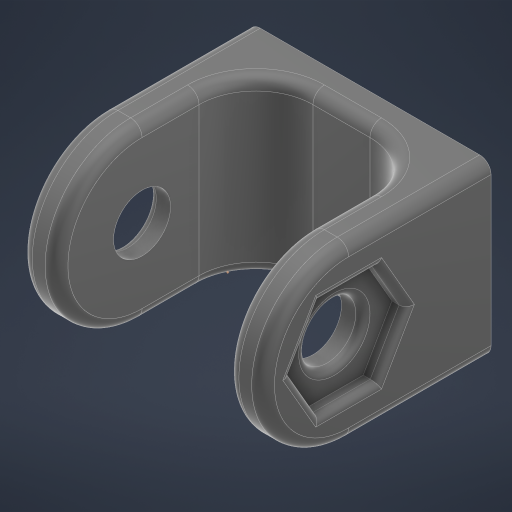
# Autodesk Inventor part: board_box_holder
Saved by Autodesk Inventor 2023 (Build 270158030, 158C)
## iProperties
Created: 2022-07-16
Part Number: board_box_holder
Material: Thermoplastic Resin
Document SubType Name: Modeling
Designer: Norbert Ligas
Density: 1.28 g/cm^3
Appearance: Smooth - Black
bar_holder_bar_diameter: 8,000 mm
bar_holder_wall_thickness: 2,000 mm
bar_holder_holder_depth: 20,000 mm
bar_holder_holder_length: 22,000 mm
bar_holder_screw_diameter: 4,000 mm
bar_holder_screw_to_bar_distance: 0,500 mm
nut_width: 7,000 mm
screw_head_diameter: 7,000 mm
bar_connector_width: 2,500 mm
bar_connector_screw_depth: 1,000 mm
bar_connector_bar_holder_width: 12,000 mm
bar_connector_length_from_screw_center_to_edge: 6,000 mm
bar_connector_min_length_from_screw_center_to_box: 6,000 mm
bar_connector_min_length_from_screw_center_to_box_margin: 2,000 mm
bar_connector_length_from_screw_center_to_box: 8,000 mm
d32: 12,000 mm
d33: 2,500 mm
d35: 6,000 mm
d36: 8,000 mm
d37: 0,00 deg
d38: 0,00 deg
d40: 0,00 deg
d41: 4,000 mm
d43: 0,00 deg
d44: 7,000 mm
d45: 1,000 mm
d46: 0,00 deg
d47: 7,000 mm
d48: 1,000 mm
d49: 0,00 deg
d50: 2,000 mm
d51: 0,00 deg
d52: 4,000 mm
d53: 0,800 mm
d54: 0,500 mm
d55: 0,500 mm
d56: 0,500 mm
d57: 0,500 mm
Author: Norbert Ligas
Autodesk Inventor part; units mm, degrees
ref_plane "YZ Plane" through (0, 0, 0) normal (1, 0, 0) x (0, 1, 0)
ref_plane "XZ Plane" through (0, 0, 0) normal (0, 1, 0) x (-1, 0, 0)
ref_plane "XY Plane" through (0, 0, 0) normal (0, 0, 1) x (1, 0, 0)
sketch "Sketch8" plane through (0, 0, 0) normal (0, 0, 1) x (1, 0, 0)
  line L0 (-6, 6) -> (-8.5, 6)
  line L1 (-8.5, 6) -> (-8.5, -6)
  line L2 (-8.5, -6) -> (-6, -6)
  line L3 (-6, -6) -> (-6, 6)
  line L4 (-6, 6) -> (-8.5, -6) construction
  line L5 (-8.5, 6) -> (-6, -6) construction
  line L6 (6, -6) -> (8.5, -6)
  line L7 (8.5, -6) -> (8.5, 6)
  line L8 (8.5, 6) -> (6, 6)
  line L9 (6, 6) -> (6, -6)
  line L10 (6, -6) -> (8.5, 6) construction
  line L11 (8.5, -6) -> (6, 6) construction
  line L12 (0, 8.4) -> (0, -8.4) projected
  line L13 (-11.9, 0) -> (11.9, 0) projected
  line L14 (-6, 6) -> (6, 6) construction
  line L15 (-6, -6) -> (6, -6) construction
  point P0 (0, 0)
  point P1 (-7.25, 0)
  point P2 (7.25, 0)
  dimension "d32" = 12
  dimension "d33" = 2.5
  constraints: 28 end point, 6 parallel, 4 horizontal, 4 midpoint, 3 equal length, 2 perpendicular, 2 point on line, 1 other
  measures "d32" distance between parallel lines of L9 L3
  measures "d33" distance of L7.end L8.end
extrude "Extrusion1" add sketch "Sketch8" along normal blind 6 and the other way blind 8
sketch "Sketch9" plane through (-8.5, -6, 6) normal (-1, 0, 0) x (0, 0, 1)
  circle A0 centre (-6, 6) radius 6
  line L0 (0, 12) -> (0, 0) construction
  line L1 (0, 6) -> (-14, 6) construction
  line L2 (-14, 12) -> (-14, 0) construction
  line L3 (0, 12) -> (-14, 12) construction
  line L4 (-14, 12) -> (0, 12) projected
  line L5 (-6, 12) -> (0, 12)
  line L6 (0, 12) -> (0, 0)
  line L7 (0, 0) -> (-6, 0)
  line L8 (-14, 0) -> (0, 0) projected
  constraints: 8 end point, 3 point on line, 2 collinear, 2 midpoint, 2 point on circle, 2 tangent, 1 centre point, 1 coincident
extrude "Extrusion2" cut sketch "Sketch9" against normal through all contours L6 L7 A0 | A0 L4 L6
sketch "Sketch10" plane through (-8.5, -6, -8) normal (-1, 0, 0) x (0, 0, 1)
  line L0 (8, 6) -> (14, 6) construction
  arc A0 (8, 0) -> (8, 12) centre (8, 6) ccw construction
  line L1 (8, 6) -> (0, 6) construction
  line L2 (0, 12) -> (0, 0) construction
  circle A1 centre (8, 6) radius 2
  dimension "d41" = 4
  constraints: 4 end point, 1 centre point, 1 coincident, 1 horizontal, 1 midpoint, 1 point on circle
  measures "d41" diameter of A1
extrude "Extrusion3" cut sketch "Sketch10" against normal through all
sketch "Sketch11" plane through (-8.5, -6, -8) normal (-1, 0, 0) x (0, 0, 1)
  circle A0 centre (8, 6) radius 3.5
  dimension "d44" = 7
  constraints: 1 centre point, 1 coincident
  measures "d44" diameter of A0
extrude "Extrusion4" cut sketch "Sketch11" against normal blind 1
sketch "Sketch12" plane through (8.5, -6, -8) normal (1, 0, 0) x (0, 0, -1)
  line L0 (-3.9585, 6) -> (-5.9793, 2.5)
  line L1 (-5.9793, 2.5) -> (-10.0207, 2.5)
  line L2 (-10.0207, 2.5) -> (-12.0415, 6)
  line L3 (-12.0415, 6) -> (-10.0207, 9.5)
  line L4 (-10.0207, 9.5) -> (-5.9793, 9.5)
  line L5 (-5.9793, 9.5) -> (-3.9585, 6)
  line L6 (0, 6) -> (-14, 6) construction
  arc A0 (-8, 12) -> (-8, 0) centre (-8, 6) ccw construction
  line L7 (0, 12) -> (0, 0) construction
  dimension "d47" = 7
  constraints: 14 end point, 1 coincident, 1 horizontal, 1 midpoint, 1 point on circle, 1 point on line, 13 other
  measures "d47" distance between parallel lines of L1 L4
extrude "Extrusion5" cut sketch "Sketch12" against normal blind 1
sketch "Sketch13" plane through (0, 0, -8) normal (0, 0, -1) x (-1, 0, 0)
  line L0 (-8.5, 6) -> (-8.5, -6) projected
  line L1 (-6, 6) -> (-8.5, 6) projected
  line L2 (8.5, -6) -> (8.5, 6) projected
  line L3 (-8.5, 6) -> (8.5, 6)
  line L4 (8.5, 6) -> (8.5, -6)
  line L5 (8.5, -6) -> (-8.5, -6)
  line L6 (-8.5, -6) -> (-8.5, 6)
  point P0 (0, 0)
  constraints: 8 end point, 2 parallel, 1 horizontal, 1 perpendicular
extrude "Extrusion6" add sketch "Sketch13" along normal blind 2
fillet "Fillet1" radius 4 2 edges at (-6, 0, -8) (6, 0, -8)
fillet "Fillet2" radius 0.8 13 edges at (6, 6, -2) (6, 0, 6) (6, -6, -2) (0, -6, -8) (-6, -6, -2) (-6, 0, 6) (-6, 6, -2) (-8.5, 6, -5) (-8.5, -6, -5) (-8.5, 0, 6) (8.5, -6, -5) (8.5, 6, -5) (8.5, 0, 6)
fillet "Fillet3" radius 0.5 1 edges at (7.5, 0, -2)
fillet "Fillet4" radius 0.5 1 edges at (-7.5, 0, -2)
fillet "Fillet5" radius 0.5 6 edges at (8.5, -1.75, 3.0311) (8.5, 1.75, 3.0311) (8.5, 3.5, 0) (8.5, 1.75, -3.0311) (8.5, -1.75, -3.0311) (8.5, -3.5, 0)
fillet "Fillet6" radius 0.5 1 edges at (-8.5, 0, -3.5)
equation "\"d32\" = bar_connector_bar_holder_width"
equation "\"d33\" = bar_connector_width"
equation "\"d35\" = bar_connector_length_from_screw_center_to_edge"
equation "\"d36\" = bar_connector_length_from_screw_center_to_box"
equation "\"d41\" = bar_holder_screw_diameter"
equation "\"d44\" = screw_head_diameter"
equation "\"d45\" = bar_connector_screw_depth"
equation "\"d47\" = nut_width"
equation "\"d48\" = bar_connector_screw_depth"
equation "\"d50\" = bar_holder_wall_thickness"
equation "\"bar_connector_width\" = 2.5"
equation "\"bar_connector_screw_depth\" = 1"
equation "\"bar_connector_bar_holder_width\" = bar_holder_bar_diameter + 2 * bar_holder_wall_thickness"
equation "\"bar_connector_length_from_screw_center_to_edge\" = 0.5 * bar_connector_bar_holder_width"
equation "\"bar_connector_length_from_screw_center_to_box\" = 8"
equation "\"bar_holder_screw_diameter\" = 4"
equation "\"screw_head_diameter\" = 7"
equation "\"nut_width\" = 7"
equation "\"bar_holder_wall_thickness\" = 2"
equation "\"bar_holder_bar_diameter\" = 8"
body "Solid3"
